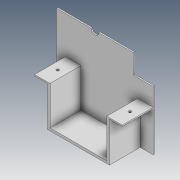
# Autodesk Inventor part: tampa
Saved by Autodesk Inventor 2021 (Build 250183000, 183)
## iProperties
Created: 2020-10-16
Part Number: tampa
Material: Genérico
Document SubType Name: Modeling
Designer: evert
Density: 1 g/cm^3
Appearance: Padrão
Author: evert
Autodesk Inventor part; units mm, degrees
ref_plane "YZ Plane" through (0, 0, 0) normal (1, 0, 0) x (0, 1, 0)
ref_plane "XZ Plane" through (0, 0, 0) normal (0, 1, 0) x (-1, 0, 0)
ref_plane "XY Plane" through (0, 0, 0) normal (0, 0, 1) x (1, 0, 0)
sketch "Esboço1" plane through (0, 0, 0) normal (0, 0, 1) x (1, 0, 0)
  line L0 (0, 0) -> (30, 0)
  line L1 (30, 0) -> (30, -36.4)
  line L2 (30, -36.4) -> (0, -36.4)
  line L3 (0, -36.4) -> (0, 0)
  dimension "d0" = 30
  dimension "d1" = 36.4
  constraints: 8 end point, 2 parallel, 1 horizontal, 1 perpendicular
  measures "d0" distance of L1.end L2.end
  measures "d1" distance of L0.end L1.end
extrude "Extrusão1" add sketch "Esboço1" along normal blind 0.5
sketch "Esboço2" plane through (0, 0, 0.5) normal (0, 0, 1) x (1, 0, 0)
  line L0 (30, 0) -> (0, 0) projected
  line L1 (0, 0) -> (15, 0)
  line L2 (15, 0) -> (15, -7.5)
  circle A0 centre (15, -7.5) radius 1.5
  dimension "d4" = 7.5
  dimension "d5" = 3
  constraints: 4 end point, 1 centre point, 1 coincident, 1 midpoint, 1 perpendicular
  measures "d4" distance of L1.end L2.end
  measures "d5" diameter of A0
extrude "Extrusão2" cut sketch "Esboço2" against normal blind 0.5
sketch "Esboço4" plane through (0, 0, 0.5) normal (0, 0, 1) x (1, 0, 0)
  line L0 (0, -36.4) -> (30, -36.4) projected
  line L1 (0, -36.4) -> (30, -36.4)
  line L2 (30, -36.4) -> (30, -37.1)
  line L3 (30, -37.1) -> (0, -37.1)
  line L4 (0, -37.1) -> (0, -36.4)
  point P0 (0, 0)
  dimension "d10" = 0.7
  constraints: 8 end point, 2 parallel, 1 horizontal, 1 perpendicular
  measures "d10" distance of L1.end L2.end
extrude "Extrusão3" add sketch "Esboço4" against normal blind 0.5
sketch "Esboço5" plane through (0, 0, 0.5) normal (0, 0, 1) x (1, 0, 0)
  line L0 (0, 0) -> (0, -37.1) projected
  line L1 (0, -37.1) -> (4, -37.1)
  line L2 (30, -37.1) -> (0, -37.1) projected
  line L3 (30, -37.1) -> (30, 0) projected
  line L4 (30, -37.1) -> (26, -37.1)
  line L5 (30, -37.1) -> (35.5, -37.1)
  line L6 (35.5, -37.1) -> (35.5, -17.1)
  line L7 (35.5, -17.1) -> (30, -17.1)
  dimension "d13" = 4
  dimension "d14" = 4
  dimension "d15" = 5.5
  dimension "d16" = 20
  constraints: 10 end point, 3 point on line, 2 perpendicular, 1 horizontal
  measures "d13" distance of L0.end L1.end
  measures "d14" distance of L2.start L4.end
  measures "d15" distance of L2.start L5.end
  measures "d16" distance of L5.end L6.end
extrude "Extrusão4" add sketch "Esboço5" against normal blind 0.5
sketch "Esboço6" plane through (0, 0, 0.5) normal (0, 0, 1) x (1, 0, 0)
  line L0 (35.5, -37.1) -> (0, -37.1) projected
  line L1 (0, -37.1) -> (9.5, -37.1)
  line L2 (35.5, -37.1) -> (31.6, -37.1)
  line L3 (35.5, -37.1) -> (36.5, -37.1)
  line L4 (36.5, -37.1) -> (36.5, -11.1125)
  line L5 (36.5, -11.1125) -> (35.5, -11.1125)
  line L6 (35.5, -11.1125) -> (35.5, -37.1)
  line L7 (30, -17.1) -> (30, 0) projected
  line L8 (30, -17.1) -> (30, -15.0997)
  line L9 (30, -15.0997) -> (36.5, -15.0997)
  line L10 (30, -17.1) -> (35.5, -17.1) projected
  line L11 (30, -17.1) -> (35.5, -17.1)
  line L12 (30, -15.0997) -> (36.5, -15.0997)
  point P0 (0, 0)
  dimension "d19" = 9.5
  dimension "d20" = 3.9
  dimension "d21" = 1
  constraints: 20 end point, 4 point on line, 3 equal length, 2 horizontal, 2 perpendicular
  measures "d19" distance of L0.end L1.end
  measures "d20" distance of L0.start L2.end
  measures "d21" distance of L5.end L4.end
extrude "Extrusão5" add sketch "Esboço6" against normal blind 0.5 contours L6 L9 L4 L3 | L10 L7 L9 L6
sketch "Esboço7" plane through (0, 0, 0.5) normal (0, 0, 1) x (1, 0, 0)
  line L0 (36.5, -37.1) -> (0, -37.1) projected
  line L1 (0, -37.1) -> (9.5, -37.1)
  line L2 (36.5, -37.1) -> (31.6, -37.1)
  line L3 (31.6, -37.1) -> (31.6, -20.6)
  line L4 (9.5, -37.1) -> (9.5, -20.6)
  line L5 (8.5, -20.6) -> (8.5, -37.1)
  line L6 (32.6, -20.6) -> (32.6, -37.1)
  line L7 (31.6, -20.6) -> (31.6, -20.1)
  line L8 (31.6, -20.1) -> (32.6, -20.1)
  line L9 (32.6, -20.1) -> (32.6, -20.6375)
  line L10 (9.5, -20.6) -> (9.5, -20.1)
  line L11 (9.5, -20.1) -> (8.5, -20.1)
  line L12 (8.5, -20.1) -> (8.5, -20.8548)
  line L13 (8.5, -37.1) -> (32.6, -37.1)
  line L14 (32.6, -37.1) -> (32.6, -36.6)
  line L15 (8.5, -37.1) -> (8.5, -36.6)
  point P0 (0, 0)
  dimension "d24" = 9.5
  dimension "d25" = 4.9
  dimension "d26" = 16.5
  dimension "d27" = 1
  dimension "d28" = 1
  dimension "d29" = 0.5
  dimension "d30" = 0.5
  dimension "d31" = 0.5
  constraints: 30 end point, 8 point on line, 4 perpendicular, 4 vertical, 2 collinear
  measures "d24" distance of L0.end L1.end
  measures "d25" distance of L0.start L2.end
  measures "d26" distance of L2.end L3.end
  measures "d27" distance of L4.end L5.start
  measures "d28" distance of L3.end L6.start
  measures "d29" distance of L3.end L7.end
  measures "d30" distance of L4.end L10.end
  measures "d31" distance of L6.end L14.end
extrude "Extrusão6" add sketch "Esboço7" along normal blind 12
sketch "Esboço8" plane through (0, 0, 0.5) normal (0, 0, 1) x (1, 0, 0)
  line L0 (0, 0) -> (0, -37.1) projected
  line L1 (0, -37.1) -> (36.5125, -37.1)
  line L2 (36.5125, -37.1) -> (36.5125, -38.1)
  line L3 (36.5125, -38.1) -> (0, -38.1)
  line L4 (0, -38.1) -> (0, -37.1)
  constraints: 8 end point, 2 parallel, 1 horizontal, 1 perpendicular
extrude "Extrusão7" add sketch "Esboço8" against normal blind 0.5
sketch "Esboço9" plane through (0, 0, 0.5) normal (0, 0, 1) x (1, 0, 0)
  line L0 (8.5, -37.1) -> (9.5, -37.1) projected
  line L1 (8.5, -37.1) -> (8.5, -38.1)
  line L2 (8.5, -38.1) -> (32.6, -38.1)
  line L3 (0, -38.1) -> (36.5125, -38.1) projected
  line L4 (31.6, -37.1) -> (32.6, -37.1) projected
  line L5 (32.6, -37.1) -> (32.6, -38.1)
  line L6 (32.6165, -37.1) -> (8.5, -37.1)
  point P0 (0, 0)
  constraints: 8 end point, 2 perpendicular, 1 point on line, 1 vertical
extrude "Extrusão8" add sketch "Esboço9" along normal blind 12
sketch "Esboço10" plane through (0, 0, 12.5) normal (0, 0, 1) x (1, 0, 0)
  line L0 (9.5, -20.1) -> (8.5, -20.1) projected
  line L1 (9.5, -37.1) -> (9.5, -20.1) projected
  line L2 (8.5, -20.1) -> (9.5, -20.1)
  line L3 (9.5, -20.1) -> (9.5, -22.1)
  line L4 (9.5, -22.1) -> (8.5, -22.1)
  line L5 (8.5, -22.1) -> (8.5, -20.1)
  line L6 (32.6, -20.1) -> (31.6, -20.1) projected
  line L7 (32.6, -38.1) -> (32.6, -20.1) projected
  line L8 (31.6, -20.1) -> (32.6, -20.1)
  line L9 (32.6, -20.1) -> (32.6, -22.1)
  line L10 (32.6, -22.1) -> (31.6, -22.1)
  line L11 (31.6, -22.1) -> (31.6, -20.1)
  point P0 (0, 0)
  dimension "d38" = 2
  constraints: 16 end point, 4 parallel, 2 horizontal, 2 perpendicular, 2 point on line
  measures "d38" distance of L4.end L0.end
extrude "Extrusão9" cut sketch "Esboço10" against normal blind 12
sketch "Esboço11" plane through (8.5, -38.1, 0.5) normal (-1, 0, 0) x (0, 0, 1)
  line L0 (12, 16) -> (0, 16) projected
  line L1 (12, 16) -> (12, 0) projected
  line L2 (0, 16) -> (12, 16)
  line L3 (12, 16) -> (12, 15.5)
  line L4 (12, 15.5) -> (0, 15.5)
  line L5 (0, 15.5) -> (0, 16)
  point P0 (-0.5, 38.1)
  dimension "d41" = 0.5
  constraints: 8 end point, 2 parallel, 1 horizontal, 1 perpendicular, 1 point on line
  measures "d41" distance of L4.end L0.end
extrude "Extrusão10" add sketch "Esboço11" along normal blind 5
sketch "Esboço12" plane through (32.6, -38.1, 12.5) normal (1, 0, 0) x (0, 0, -1)
  line L0 (12, 16) -> (0, 16) projected
  line L1 (12, 15.5) -> (0, 15.5) projected
  line L2 (0, 16) -> (12, 16)
  line L3 (12, 16) -> (12, 15.5)
  line L4 (12, 15.5) -> (0, 15.5)
  line L5 (0, 15.5) -> (0, 16)
  point P0 (12.5, 38.1)
  constraints: 8 end point, 2 parallel, 1 horizontal, 1 perpendicular
extrude "Extrusão11" add sketch "Esboço12" along normal blind 5
sketch "Esboço13" plane through (0, 0, 0.5) normal (0, 0, 1) x (1, 0, 0)
  circle A0 centre (15, -7.5) radius 1.5 projected
  line L0 (15, -7.5) -> (30, -7.5)
  line L1 (30, -15.0997) -> (30, 0) projected
  line L2 (15, -7.5) -> (0, -7.5)
  line L3 (0, -38.1) -> (0, 0) projected
  line L4 (0, 0) -> (30, 0)
  line L5 (30, 0) -> (0, 0) projected
  line L6 (30, 0) -> (30, -7.5)
  line L7 (0, -7.5) -> (0, 0)
  point P0 (13.5, -7.5)
  point P1 (16.5, -7.5)
  constraints: 10 end point, 3 point on line, 2 collinear, 2 horizontal
extrude "Extrusão12" cut sketch "Esboço13" against normal blind 5 contours A0 L2 L3 L4 L1 L0
sketch "Esboço14" plane through (31.6, -22.1, 12.5) normal (0, 1, 0) x (1, 0, 0)
  line L0 (-22.1, 0) -> (-28.1, 0) projected
  line L1 (-28.1, 0) -> (-25.1, 0)
  line L2 (-25.1, 0) -> (-25.1, 6)
  line L3 (-22.1, 12) -> (-28.1, 12) projected
  line L4 (6, 12) -> (6, 0) projected
  line L5 (6, 0) -> (3, 0)
  line L6 (6, 0) -> (0, 0) projected
  line L7 (3, 0) -> (3, 6)
  circle A0 centre (-25.1, 6) radius 0.5
  circle A1 centre (3, 6) radius 0.5
  point P0 (-31.6, 12.5)
  dimension "d48" = 6
  dimension "d49" = 1
  dimension "d50" = 1
  constraints: 8 end point, 2 centre point, 2 coincident, 2 midpoint, 1 perpendicular, 1 vertical
  measures "d48" distance of L1.end L2.end
  measures "d49" diameter of A0
  measures "d50" diameter of A1
extrude "Extrusão13" cut sketch "Esboço14" against normal blind 5
sketch "Esboço15" plane through (37.6, -22.1, 0.5) normal (0, 0, -1) x (-1, 0, 0)
  line L0 (7.6, 7.0003) -> (1.1, 7.0003) projected
  line L1 (1.1, 7.0003) -> (0, 7.0003)
  line L2 (0, 7.0003) -> (0, -16)
  line L3 (1.0875, -15) -> (1.0875, -16) projected
  line L4 (0, -16) -> (1.0875, -16)
  line L5 (1.1, 7.0003) -> (1.8775, 7.0003)
  line L6 (1.8775, 7.0003) -> (1.8775, -16)
  line L7 (1.0875, -16) -> (37.6, -16) projected
  line L8 (0, -16) -> (1.8775, -16)
  point P0 (37.6, 22.1)
  constraints: 12 end point, 4 perpendicular, 2 point on line, 1 horizontal
extrude "Extrusão14" add sketch "Esboço15" along normal blind 0.5
